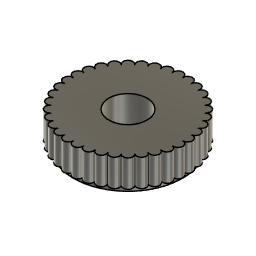
Screw Knob v1 (Autodesk Fusion 360 design; units mm, degrees)
Autodesk Fusion 360 part; units mm, degrees
sketch "Schizzo1" plane through (0, 0, 0) normal (0, 0, 1) x (1, 0, 0)
  circle A0 centre (30, 20) radius 10
  circle A1 centre (30, 20) radius 1.9
  circle A2 centre (30, 20) radius 3.5
  dimension "d1" = 20
  dimension "d2" = 3.8
  dimension "d3" = 7
  constraint concentric A0 A1
  constraint concentric A1 A2
  measures "d1" diameter of A0
  measures "d2" diameter of A1
  measures "d3" diameter of A2
extrude "Estrusione1" add sketch "Schizzo1" along normal blind 6 contours A0
extrude "Estrusione2" add sketch "Schizzo1" along normal blind 1 contours A2
sketch "Schizzo2" plane through (0, 0, 6) normal (0, 0, 1) x (-1, 0, 0)
  circle A0 centre (-30, -20) radius 3.5
  circle A1 centre (-30, -20) radius 10
  circle A2 centre (-30, -20) radius 10.0501 construction
  line L0 (-30, -20) -> (-30, -30.0501) construction
  line L1 (-30, -20) -> (-31.7452, -29.8974) construction
  arc A3 (-31.7452, -29.8974) -> (-30, -30.0501) centre (-30.881, -30.0696) ccw
  line L2 (-30, -30.0501) -> (-31.7452, -29.8974)
  arc A4 (-30, -30.0501) -> (-28.2548, -29.8974) centre (-29.119, -30.0696) ccw
  line L3 (-28.2548, -29.8974) -> (-30, -30.0501)
  arc A5 (-28.2548, -29.8974) -> (-26.5627, -29.444) centre (-27.3838, -29.7637) ccw
  line L4 (-26.5627, -29.444) -> (-28.2548, -29.8974)
  arc A6 (-26.5627, -29.444) -> (-24.9749, -28.7037) centre (-25.7281, -29.1611) ccw
  line L5 (-24.9749, -28.7037) -> (-26.5627, -29.444)
  arc A7 (-24.9749, -28.7037) -> (-23.5399, -27.6988) centre (-24.2022, -28.2801) ccw
  line L6 (-23.5399, -27.6988) -> (-24.9749, -28.7037)
  arc A8 (-23.5399, -27.6988) -> (-22.3012, -26.4601) centre (-22.8525, -27.1475) ccw
  line L7 (-22.3012, -26.4601) -> (-23.5399, -27.6988)
  arc A9 (-22.3012, -26.4601) -> (-21.2963, -25.0251) centre (-21.7199, -25.7978) ccw
  line L8 (-21.2963, -25.0251) -> (-22.3012, -26.4601)
  arc A10 (-21.2963, -25.0251) -> (-20.556, -23.4373) centre (-20.8389, -24.2719) ccw
  line L9 (-20.556, -23.4373) -> (-21.2963, -25.0251)
  arc A11 (-20.556, -23.4373) -> (-20.1026, -21.7452) centre (-20.2363, -22.6162) ccw
  line L10 (-20.1026, -21.7452) -> (-20.556, -23.4373)
  arc A12 (-20.1026, -21.7452) -> (-19.9499, -20) centre (-19.9304, -20.881) ccw
  line L11 (-19.9499, -20) -> (-20.1026, -21.7452)
  arc A13 (-19.9499, -20) -> (-20.1026, -18.2548) centre (-19.9304, -19.119) ccw
  line L12 (-20.1026, -18.2548) -> (-19.9499, -20)
  arc A14 (-20.1026, -18.2548) -> (-20.556, -16.5627) centre (-20.2363, -17.3838) ccw
  line L13 (-20.556, -16.5627) -> (-20.1026, -18.2548)
  arc A15 (-20.556, -16.5627) -> (-21.2963, -14.9749) centre (-20.8389, -15.7281) ccw
  line L14 (-21.2963, -14.9749) -> (-20.556, -16.5627)
  arc A16 (-21.2963, -14.9749) -> (-22.3012, -13.5399) centre (-21.7199, -14.2022) ccw
  line L15 (-22.3012, -13.5399) -> (-21.2963, -14.9749)
  arc A17 (-22.3012, -13.5399) -> (-23.5399, -12.3012) centre (-22.8525, -12.8525) ccw
  line L16 (-23.5399, -12.3012) -> (-22.3012, -13.5399)
  arc A18 (-23.5399, -12.3012) -> (-24.9749, -11.2963) centre (-24.2022, -11.7199) ccw
  line L17 (-24.9749, -11.2963) -> (-23.5399, -12.3012)
  arc A19 (-24.9749, -11.2963) -> (-26.5627, -10.556) centre (-25.7281, -10.8389) ccw
  line L18 (-26.5627, -10.556) -> (-24.9749, -11.2963)
  arc A20 (-26.5627, -10.556) -> (-28.2548, -10.1026) centre (-27.3838, -10.2363) ccw
  line L19 (-28.2548, -10.1026) -> (-26.5627, -10.556)
  arc A21 (-28.2548, -10.1026) -> (-30, -9.9499) centre (-29.119, -9.9304) ccw
  line L20 (-30, -9.9499) -> (-28.2548, -10.1026)
  arc A22 (-30, -9.9499) -> (-31.7452, -10.1026) centre (-30.881, -9.9304) ccw
  line L21 (-31.7452, -10.1026) -> (-30, -9.9499)
  arc A23 (-31.7452, -10.1026) -> (-33.4373, -10.556) centre (-32.6162, -10.2363) ccw
  line L22 (-33.4373, -10.556) -> (-31.7452, -10.1026)
  arc A24 (-33.4373, -10.556) -> (-35.0251, -11.2963) centre (-34.2719, -10.8389) ccw
  line L23 (-35.0251, -11.2963) -> (-33.4373, -10.556)
  arc A25 (-35.0251, -11.2963) -> (-36.4601, -12.3012) centre (-35.7978, -11.7199) ccw
  line L24 (-36.4601, -12.3012) -> (-35.0251, -11.2963)
  arc A26 (-36.4601, -12.3012) -> (-37.6988, -13.5399) centre (-37.1475, -12.8525) ccw
  line L25 (-37.6988, -13.5399) -> (-36.4601, -12.3012)
  arc A27 (-37.6988, -13.5399) -> (-38.7037, -14.9749) centre (-38.2801, -14.2022) ccw
  line L26 (-38.7037, -14.9749) -> (-37.6988, -13.5399)
  arc A28 (-38.7037, -14.9749) -> (-39.444, -16.5627) centre (-39.1611, -15.7281) ccw
  line L27 (-39.444, -16.5627) -> (-38.7037, -14.9749)
  arc A29 (-39.444, -16.5627) -> (-39.8974, -18.2548) centre (-39.7637, -17.3838) ccw
  line L28 (-39.8974, -18.2548) -> (-39.444, -16.5627)
  arc A30 (-39.8974, -18.2548) -> (-40.0501, -20) centre (-40.0696, -19.119) ccw
  line L29 (-40.0501, -20) -> (-39.8974, -18.2548)
  arc A31 (-40.0501, -20) -> (-39.8974, -21.7452) centre (-40.0696, -20.881) ccw
  line L30 (-39.8974, -21.7452) -> (-40.0501, -20)
  arc A32 (-39.8974, -21.7452) -> (-39.444, -23.4373) centre (-39.7637, -22.6162) ccw
  line L31 (-39.444, -23.4373) -> (-39.8974, -21.7452)
  arc A33 (-39.444, -23.4373) -> (-38.7037, -25.0251) centre (-39.1611, -24.2719) ccw
  line L32 (-38.7037, -25.0251) -> (-39.444, -23.4373)
  arc A34 (-38.7037, -25.0251) -> (-37.6988, -26.4601) centre (-38.2801, -25.7978) ccw
  line L33 (-37.6988, -26.4601) -> (-38.7037, -25.0251)
  arc A35 (-37.6988, -26.4601) -> (-36.4601, -27.6988) centre (-37.1475, -27.1475) ccw
  line L34 (-36.4601, -27.6988) -> (-37.6988, -26.4601)
  arc A36 (-36.4601, -27.6988) -> (-35.0251, -28.7037) centre (-35.7978, -28.2801) ccw
  line L35 (-35.0251, -28.7037) -> (-36.4601, -27.6988)
  arc A37 (-35.0251, -28.7037) -> (-33.4373, -29.444) centre (-34.2719, -29.1611) ccw
  line L36 (-33.4373, -29.444) -> (-35.0251, -28.7037)
  arc A38 (-33.4373, -29.444) -> (-31.7452, -29.8974) centre (-32.6162, -29.7637) ccw
  line L37 (-31.7452, -29.8974) -> (-33.4373, -29.444)
  dimension "d8" = 10
  dimension "d10" = 360
  constraint concentric A0 A2
  constraint coincident A0.centre A1.centre
  constraint coincident A2 L0.end
  constraint vertical L0
  constraint coincident A2 L1.end
  measures "d8" angle of L0 L1
extrude "Estrusione3" add sketch "Schizzo2" 1 faces at (37.7961, 19.5032, 6) against normal blind 5 contours A1 | L2 L3 L4 L5 L6 L7 L8 L9 L10 L11 L12 L13 L14 L15 L16 L17 L18 L19 L20 L21 L22 L23 L24 L25 L26 L27 L28 L29 L30 L31 L32 L33 L34 L35 L36 L37 | A3 L2 A4 A38 | A3 A37 A38 L37 | A3 A4 L3 A5 | A36 A37 L36 A38 | A4 A5 L4 A6 | A35 A36 L35 A37 | A5 A6 L5 A7 | A34 A35 L34 A36 | A6 A7 L6 A8 | A33 A34 L33 A35 | A7 A8 L7 A9 | A32 A33 L32 A34 | A8 A9 L8 A10 | A31 A32 L31 A33 | A9 A10 L9 A11 | A30 A31 L30 A32 | A10 A11 L10 A12 | A29 A30 L29 A31 | A11 A12 L11 A13 | A28 A29 L28 A30 | A12 A13 L12 A14 | A27 A28 L27 A29 | A13 A14 L13 A15 | A26 A27 L26 A28 | A14 A15 L14 A16 | A25 A26 L25 A27 | A15 A16 L15 A17 | A24 A25 L24 A26 | A16 A17 L16 A18 | A23 A24 L23 A25 | A17 A18 L17 A19 | A22 A23 L22 A24 | A18 A19 L18 A20 | A21 A22 L21 A23 | A19 A20 L19 A21 | A20 A21 L20 A22
